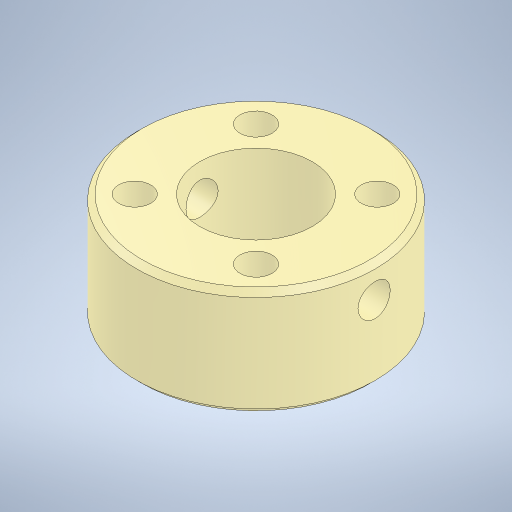
# Autodesk Inventor part: Hub Adapter
Saved by Autodesk Inventor 2023.4 (Build 274418000, 418)
## iProperties
Created: 2024-05-15
Part Number: Hub Adapter
Material: Nylon 6/6
Document SubType Name: Modeling
Designer: Nathan Cai
Density: 1.13 g/cm^3
Appearance: Nylon 6
Author: Nathan Cai
Autodesk Inventor part; units mm, degrees
ref_plane "YZ Plane" through (0, 0, 0) normal (1, 0, 0) x (0, 1, 0)
ref_plane "XZ Plane" through (0, 0, 0) normal (0, 1, 0) x (-1, 0, 0)
ref_plane "XY Plane" through (0, 0, 0) normal (0, 0, 1) x (1, 0, 0)
sketch "Sketch1" plane through (0, 0, 0) normal (0, 1, 0) x (-1, 0, 0)
  circle A0 centre (0, 0) radius 11.1125
  circle A1 centre (0, 0) radius 8 construction
  line L0 (0, 0) -> (0, -8) construction
  line L1 (0, 0) -> (5.6569, -5.6569) construction
  circle A2 centre (5.6569, -5.6569) radius 1.5
  circle A3 centre (5.6569, 5.6569) radius 1.5
  circle A4 centre (-5.6569, 5.6569) radius 1.5
  circle A5 centre (-5.6569, -5.6569) radius 1.5
  circle A6 centre (0, 0) radius 5.25
  dimension "d0" = 22.225
  dimension "d1" = 16
  dimension "d2" = 45
  dimension "d3" = 3
  dimension "d6" = 360
  dimension "d8" = 10.5
  constraints: 7 centre point, 4 coincident, 4 end point, 2 point on circle, 1 vertical, 9 other
  measures "d0" diameter of A0
  measures "d1" diameter of A1
  measures "d2" angle of L1 L0
  measures "d3" diameter of A2
  measures "d8" diameter of A6
extrude "Extrusion1" add sketch "Sketch1" along normal blind 10
sketch "Sketch2" plane through (0, 0, 0) normal (1, 0, 0) x (0, 1, 0)
  line L0 (10, -11.1125) -> (10, 11.1125) projected
  line L1 (10, 0) -> (0, 0) construction
  circle A0 centre (7, 0) radius 1.5
  line L2 (0, -11.1125) -> (0, 11.1125) projected
  dimension "d11" = 3
  dimension "d12" = 7
  constraints: 2 end point, 1 centre point, 1 horizontal, 1 midpoint, 1 point on line
  measures "d11" diameter of A0
  measures "d12" distance from line of L2 A0.centre
extrude "Extrusion2" cut sketch "Sketch2" along normal through all both and the other way through all
chamfer "Chamfer1" distance 0.5 angle 45 1 edges at (5.25, 0, 0)
chamfer "Chamfer2" distance 0.5 angle 45 2 edges at (11.1125, 10, 0) (11.1125, 0, 0)
body "Solid1"
